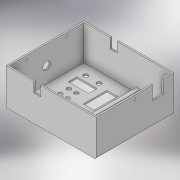
# Autodesk Inventor part: case
Saved by Autodesk Inventor 2019 (Build 230136000, 136)
## iProperties
Created: 2020-05-08
Part Number: case
Material: Generic
Document SubType Name: Modeling
Designer: Mateusz
Density: 1 g/cm^3
Appearance: Default
Author: Mateusz
Autodesk Inventor part; units mm, degrees
ref_plane "YZ Plane" through (0, 0, 0) normal (1, 0, 0) x (0, 1, 0)
ref_plane "XZ Plane" through (0, 0, 0) normal (0, 1, 0) x (-1, 0, 0)
ref_plane "XY Plane" through (0, 0, 0) normal (0, 0, 1) x (1, 0, 0)
sketch "Sketch1" plane through (0, 0, 0) normal (0, 1, 0) x (-1, 0, 0)
  line L0 (0, 0) -> (0, 98.75)
  line L1 (0, 98.75) -> (114.73, 98.75)
  line L2 (114.73, 98.75) -> (114.73, 0)
  line L3 (114.73, 0) -> (0, 0)
  line L4 (0, 98.75) -> (0, 90.47)
  line L5 (0, 0) -> (0, 6.72)
  line L6 (114.73, 0) -> (114.73, 9.87)
  line L7 (-2, 0) -> (-2, 98.75)
  line L8 (-2, 98.75) -> (-2, 100.75)
  line L9 (-2, 100.75) -> (114.73, 100.75)
  line L10 (114.73, 100.75) -> (116.73, 100.75)
  line L11 (116.73, 100.75) -> (116.73, 0)
  line L12 (116.73, 0) -> (116.73, -2)
  line L13 (116.73, -2) -> (-2, -2)
  line L14 (-2, -2) -> (-2, 0)
  dimension "d11" = 2
  dimension "d12" = 2
  dimension "d13" = 2
  dimension "d14" = 2
  constraints: 30 end point, 7 point on line, 6 perpendicular, 1 horizontal, 1 vertical
  measures "d11" distance of L0.start L7.start
  measures "d12" distance of L7.end L8.end
  measures "d13" distance of L9.end L10.end
  measures "d14" distance of L11.end L12.end
extrude "Extrusion1" add sketch "Sketch1" along normal blind 2 contours L0 L1 L2 L3 | L7 L8 L9 L10 L11 L12 L13 L14
extrude "Extrusion9" add sketch "Sketch1" along normal blind 48
sketch "Sketch11" plane through (0, 2, 0) normal (0, 1, 0) x (1, 0, 0)
  circle A0 centre (-60.73, -74.125) radius 3.75 projected
  line L0 (-68.73, -5.5) -> (-68.73, -51.875) projected
  line L1 (-68.73, -5.5) -> (-52.73, -5.5) projected
  line L2 (-68.73, -51.875) -> (-52.73, -51.875) projected
  line L3 (-52.73, -51.875) -> (-52.73, -5.5) projected
  line L4 (-68.53, -92.03) -> (-68.53, -66.625) projected
  line L5 (-68.53, -66.625) -> (-53.65, -66.625) projected
  line L6 (-53.65, -66.625) -> (-53.65, -92.03) projected
  line L7 (-53.65, -92.03) -> (-45.73, -92.03) projected
  line L8 (-45.73, -92.03) -> (-45.73, -5.5) projected
  line L9 (-48.73, -5.5) -> (-45.73, -5.5) projected
  line L10 (-48.73, -5.5) -> (-48.73, -55.875) projected
  line L11 (-48.73, -55.875) -> (-72.73, -55.875) projected
  line L12 (-72.73, -55.875) -> (-72.73, -5.5) projected
  line L13 (-75.73, -5.5) -> (-72.73, -5.5) projected
  line L14 (-75.73, -5.5) -> (-75.73, -17.875) projected
  line L15 (-75.73, -17.875) -> (-85.89, -17.875) projected
  line L16 (-85.89, -17.875) -> (-85.89, -5.5) projected
  line L17 (-85.89, -5.5) -> (-93.51, -5.5) projected
  line L18 (-93.51, -5.5) -> (-93.51, -17.875) projected
  line L19 (-93.51, -17.875) -> (-103.67, -17.875) projected
  line L20 (-103.67, -17.875) -> (-103.67, -5.5) projected
  line L21 (-111.73, -5.5) -> (-103.67, -5.5) projected
  line L22 (-111.73, -5.5) -> (-111.73, -93.25) projected
  line L23 (-111.73, -93.25) -> (-103.67, -93.25) projected
  line L24 (-103.67, -93.25) -> (-103.67, -80.875) projected
  line L25 (-103.67, -80.875) -> (-93.51, -80.875) projected
  line L26 (-93.51, -80.875) -> (-93.51, -92.03) projected
  line L27 (-93.51, -92.03) -> (-85.89, -92.03) projected
  line L28 (-85.89, -92.03) -> (-85.89, -80.875) projected
  line L29 (-85.89, -80.875) -> (-75.73, -80.875) projected
  line L30 (-75.73, -80.875) -> (-75.73, -92.03) projected
  line L31 (-75.73, -92.03) -> (-68.53, -92.03) projected
  line L32 (-56.73, -92.03) -> (-56.73, -81.625) projected
  line L33 (-56.73, -81.625) -> (-64.73, -81.625) projected
  line L34 (-64.73, -81.625) -> (-64.73, -92.03) projected
  line L35 (-64.73, -92.03) -> (-56.73, -92.03) projected
  circle A1 centre (-98.59, -84.875) radius 1.65 projected
  circle A2 centre (-80.81, -84.875) radius 1.65 projected
  circle A3 centre (-60.73, -74.125) radius 3.75 projected
  line L36 (-114.73, -98.25) -> (-114.73, -0.5) projected
  line L37 (-114.73, -0.5) -> (-42.73, -0.5) projected
  line L38 (-42.73, -0.5) -> (-42.73, -98.25) projected
  line L39 (-114.73, -98.25) -> (-42.73, -98.25) projected
  circle A4 centre (-70.73, -23.875) radius 1 projected
  circle A5 centre (-50.73, -23.875) radius 1 projected
  circle A6 centre (-60.73, -53.875) radius 1 projected
  circle A7 centre (-80.81, -13.875) radius 1.65 projected
  circle A8 centre (-98.59, -13.875) radius 1.65 projected
  line L40 (-68.73, -5.5) -> (-68.73, -51.875) projected
  line L41 (-68.73, -51.875) -> (-52.73, -51.875) projected
  line L42 (-52.73, -51.875) -> (-52.73, -5.5) projected
  line L43 (-68.73, -5.5) -> (-52.73, -5.5) projected
  circle A9 centre (-60.73, -74.125) radius 7.5
  line L44 (-67.83, -47.875) -> (-53.63, -47.875)
  line L45 (-67.83, -16.5) -> (-67.83, -47.875)
  line L46 (-53.63, -47.875) -> (-53.63, -16.5)
  line L47 (-53.63, -16.5) -> (-67.83, -16.5)
  line L48 (-42.73, -98.25) -> (-39.73, -98.25)
  line L49 (-39.73, -98.25) -> (-39.73, -0.5)
  line L50 (-39.73, -0.5) -> (-42.73, -0.5)
  line L51 (-42.73, -0.5) -> (-42.73, -98.25)
  circle A10 centre (-96.54, -74.125) radius 3.25
  circle A11 centre (-84.58, -61.395) radius 2.75
  circle A12 centre (-94.53, -61.295) radius 2.75
  circle A13 centre (-94.53, -51.135) radius 2.75
  circle A14 centre (-84.58, -51.395) radius 2.75
  circle A15 centre (-94.53, -40.055) radius 2.75
  circle A16 centre (-84.58, -40.145) radius 2.75
  line L52 (-76.36, -32.405) -> (-103.04, -32.405)
  line L53 (-76.36, -32.405) -> (-76.36, -20.965)
  line L54 (-76.36, -20.965) -> (-103.04, -20.965)
  line L55 (-103.04, -20.965) -> (-103.04, -32.405)
  circle A17 centre (-98.59, -84.875) radius 3
  circle A18 centre (-80.81, -84.875) radius 3
  circle A19 centre (-98.59, -13.875) radius 3
  circle A20 centre (-80.81, -13.875) radius 3
  circle A21 centre (-82.79, -74.125) radius 3.25
  point P0 (0, 0)
  dimension "d49" = 15
  dimension "d56" = 3
  dimension "d109" = 11.44
  dimension "d127" = 6
  dimension "d128" = 6
  dimension "d129" = 6
  dimension "d130" = 6
  dimension "d191" = 6.5
  constraints: 24 end point, 13 centre point, 5 coincident, 4 perpendicular, 2 horizontal, 1 parallel, 1 vertical
  measures "d49" diameter of A9
  measures "d56" distance of L38.end L48.end
  measures "d109" distance of L52.start L53.end
  measures "d127" diameter of A17
  measures "d128" diameter of A18
  measures "d129" diameter of A19
  measures "d130" diameter of A20
  measures "d191" diameter of A21
extrude "Extrusion10" cut sketch "Sketch11" against normal blind 10 contours A0 | A9 L6 | A9 L6 | L45 L47 L46 L44
extrude "Extrusion11" add sketch "Sketch11" along normal blind 7 contours L38 L50 L49 L48
sketch "Sketch12" plane through (-42.73, 2, 0.5) normal (-1, 0, 0) x (0, 0, 1)
  line L0 (97.75, 7) -> (97.75, 5)
  line L1 (97.75, 0) -> (97.75, 7) projected
  line L2 (97.75, 7) -> (0, 7) projected
  line L3 (0, 7) -> (0, 5)
  line L4 (0, 0) -> (0, 7) projected
  line L5 (0, 5) -> (97.75, 5)
  line L6 (97.75, 7) -> (0, 7)
  point P0 (-0.5, -2)
  dimension "d61" = 2
  dimension "d62" = 2
  constraints: 8 end point, 2 point on line
  measures "d61" distance of L0.start L0.end
  measures "d62" distance of L2.end L3.end
extrude "Extrusion12" add sketch "Sketch12" along normal blind 2
extrude "Extrusion13" cut sketch "Sketch11" against normal blind 5 contours A1 | A2 | A7 | A8 | A10 | A11 | A12 | A13 | A14 | A15 | A16 | A21
extrude "Extrusion14" cut sketch "Sketch11" against normal blind 5 contours L52 L55 L54 L53
sketch "Sketch13" plane through (2, 0, 100.75) normal (1, 0, 0) x (0, 0, -1)
  line L0 (88.25, 41) -> (88.75, 41)
  line L1 (88.75, 41) -> (88.75, 48)
  line L2 (88.75, 48) -> (74.75, 48)
  line L3 (74.75, 48) -> (74.75, 41)
  line L4 (74.75, 41) -> (74.75, 30)
  line L5 (74.75, 30) -> (88.5, 30)
  line L6 (88.5, 30) -> (88.75, 30)
  line L7 (88.75, 30) -> (88.75, 41)
  point P0 (100.75, 0)
  point P1 (102.75, 48)
  dimension "d116" = 0.5
  dimension "d118" = 11
  constraints: 16 end point, 3 perpendicular, 2 point on line
  measures "d116" distance of L0.start L0.end
  measures "d118" distance of L3.end L4.end
extrude "Extrusion15" cut sketch "Sketch13" against normal blind 5
sketch "Sketch14" plane through (-116.73, 0, 100.75) normal (0, 0, 1) x (1, 0, 0)
  line L0 (0, 0) -> (0, 48) projected
  line L1 (0, 48) -> (2, 48)
  line L2 (2, 48) -> (36, 48)
  line L3 (2, 48) -> (116.73, 48) projected
  line L4 (36, 48) -> (45, 48)
  line L5 (36, 48) -> (36.715, 48)
  line L6 (0, 48) -> (118.73, 48) projected
  line L7 (36.715, 48) -> (36.715, 35)
  line L8 (45, 48) -> (45.715, 48)
  line L9 (45.715, 48) -> (45.715, 35)
  line L10 (45.715, 35) -> (45, 35)
  line L11 (36.715, 35) -> (45, 35)
  point P0 (116.73, 0)
  dimension "d121" = 2
  dimension "d122" = 34
  dimension "d123" = 9
  dimension "d124" = 13
  dimension "d196" = 0.715
  dimension "d197" = 0.715
  constraints: 18 end point, 4 point on line, 2 perpendicular, 1 collinear, 1 horizontal
  measures "d121" distance of L0.end L1.end
  measures "d122" distance of L1.end L2.end
  measures "d123" distance of L2.end L4.end
  measures "d124" distance of L4.end L10.end
  measures "d196" distance of L2.end L5.end
  measures "d197" distance of L4.end L8.end
extrude "Extrusion16" cut sketch "Sketch14" against normal blind 120
extrude "Extrusion17" add sketch "Sketch11" along normal blind 2 contours A17 | A18 | A19 | A20
sketch "Sketch15" plane through (0, 0, 0) normal (0, -1, 0) x (1, 0, 0)
  line L0 (-2, 12) -> (-2, 26)
  line L1 (-2, 26) -> (-12, 26)
  line L2 (-12, 26) -> (-12, 12)
  line L3 (-12, 12) -> (-2, 12)
  point P0 (0, 0)
  point P1 (2, 12)
  dimension "d134" = 10
  constraints: 8 end point, 3 perpendicular
  measures "d134" distance of L0.end L1.end
extrude "Extrusion18" cut sketch "Sketch15" against normal blind 0.5
sketch "Sketch16" plane through (-116.73, 0, -2) normal (-1, 0, 0) x (0, 0, 1)
  line L0 (2, 48) -> (0, 48) projected
  line L1 (0, 48) -> (20, 48)
  line L2 (100.75, 48) -> (2, 48) projected
  line L3 (20, 48) -> (20, 43)
  line L4 (20, 43) -> (30, 43)
  line L5 (30, 43) -> (25, 43)
  circle A0 centre (25, 43) radius 1.45
  line L6 (102.75, 48) -> (82.75, 48)
  line L7 (28, 48) -> (100.75, 48) projected
  line L8 (82.75, 48) -> (82.75, 43)
  line L9 (82.75, 43) -> (77.75, 43)
  circle A1 centre (77.75, 43) radius 1.45
  point P0 (2, 0)
  dimension "d137" = 20
  dimension "d138" = 5
  dimension "d139" = 10
  dimension "d140" = 2.9
  dimension "d141" = 20
  dimension "d142" = 5
  dimension "d143" = 5
  dimension "d144" = 2.9
  constraints: 14 end point, 3 perpendicular, 2 centre point, 2 coincident, 2 point on line, 1 midpoint, 1 vertical
  measures "d137" distance of L0.end L1.end
  measures "d138" distance of L1.end L3.end
  measures "d139" distance of L3.end L4.end
  measures "d140" diameter of A0
  measures "d141" distance of L6.start L6.end
  measures "d142" distance of L6.end L8.end
  measures "d143" distance of L8.end L9.end
  measures "d144" diameter of A1
extrude "Extrusion19" cut sketch "Sketch16" against normal blind 3
sketch "Sketch17" plane through (2, 0, 100.75) normal (1, 0, 0) x (0, 0, -1)
  circle A0 centre (51.375, 43) radius 1.45
  point P0 (100.75, 0)
  point P1 (0, 48)
  constraints: 1 centre point
extrude "Extrusion20" cut sketch "Sketch17" against normal blind 3
sketch "Sketch18" plane through (0, 0, 0) normal (0, -1, 0) x (1, 0, 0)
  line L0 (-99.53, 40.055) -> (-99.53, 61.295)
  line L1 (-99.53, 61.295) -> (-99.53, 63.795)
  line L2 (-99.53, 63.795) -> (-103.53, 63.795)
  line L3 (-103.53, 63.795) -> (-103.53, 40.055)
  line L4 (-103.53, 40.055) -> (-103.53, 37.555)
  line L5 (-103.53, 37.555) -> (-99.53, 37.555)
  line L6 (-99.53, 37.555) -> (-99.53, 40.055)
  line L7 (-79.58, 61.395) -> (-79.58, 63.895)
  line L8 (-79.58, 63.895) -> (-75.58, 63.895)
  line L9 (-75.58, 63.895) -> (-75.58, 40.055)
  line L10 (-75.58, 40.055) -> (-75.58, 37.555)
  line L11 (-75.58, 37.555) -> (-79.58, 37.555)
  line L12 (-79.58, 37.555) -> (-79.58, 63.895)
  line L13 (-103.04, 20.965) -> (-76.36, 20.965) projected
  line L14 (-103.04, 20.965) -> (-105.04, 20.965)
  line L15 (-105.04, 20.965) -> (-105.04, 32.405)
  line L16 (-103.04, 32.405) -> (-76.36, 32.405) projected
  line L17 (-105.04, 32.405) -> (-109.04, 32.405)
  line L18 (-109.04, 32.405) -> (-109.04, 20.965)
  line L19 (-109.04, 20.965) -> (-105.04, 20.965)
  circle A0 centre (-96.54, 74.125) radius 3.25 projected
  line L20 (-96.54, 74.125) -> (-101.54, 74.125)
  line L21 (-101.54, 74.125) -> (-101.54, 78.125)
  line L22 (-101.54, 78.125) -> (-105.54, 78.125)
  line L23 (-105.54, 78.125) -> (-105.54, 70.125)
  line L24 (-105.54, 70.125) -> (-101.54, 70.125)
  line L25 (-101.54, 70.125) -> (-101.54, 74.125)
  line L26 (-70.73, 74.125) -> (-70.73, 78.125)
  line L27 (-70.73, 78.125) -> (-74.73, 78.125)
  line L28 (-74.73, 78.125) -> (-74.73, 70.125)
  line L29 (-74.73, 70.125) -> (-70.73, 70.125)
  line L30 (-70.73, 74.125) -> (-70.73, 70.125)
  line L31 (-69.83, 47.875) -> (-69.83, 16.5)
  line L32 (-69.83, 16.5) -> (-73.83, 16.5)
  line L33 (-73.83, 16.5) -> (-73.83, 47.875)
  line L34 (-73.83, 47.875) -> (-69.83, 47.875)
  circle A1 centre (-82.79, 74.125) radius 3.25 projected
  line L35 (-82.79, 74.125) -> (-87.79, 74.125)
  line L36 (-87.79, 74.125) -> (-87.79, 78.125)
  line L37 (-87.79, 78.125) -> (-91.79, 78.125)
  line L38 (-91.79, 78.125) -> (-91.79, 70.125)
  line L39 (-91.79, 70.125) -> (-87.79, 70.125)
  line L40 (-87.79, 70.125) -> (-87.79, 74.125)
  point P0 (0, 0)
  point P1 (-94.53, 40.055)
  point P2 (-84.58, 61.395)
  point P3 (-85.81, 74.125)
  point P4 (-85.81, 78.125)
  point P5 (-89.81, 78.125)
  point P6 (-89.81, 70.125)
  point P7 (-85.81, 70.125)
  point P8 (-67.83, 47.875)
  dimension "d153" = 2.5
  dimension "d154" = 4
  dimension "d155" = 2.5
  dimension "d157" = 2.5
  dimension "d158" = 4
  dimension "d159" = 2.5
  dimension "d160" = 4
  dimension "d161" = 2
  dimension "d162" = 4
  dimension "d163" = 5
  dimension "d164" = 4
  dimension "d165" = 4
  dimension "d166" = 8
  dimension "d171" = 4
  dimension "d172" = 4
  dimension "d173" = 8
  dimension "d175" = 4
  dimension "d198" = 5
  dimension "d199" = 4
  dimension "d200" = 8
  constraints: 78 end point, 24 perpendicular, 14 point on line, 2 horizontal, 1 parallel
  measures "d153" distance of L0.end L1.end
  measures "d154" distance of L1.end L2.end
  measures "d155" distance of L3.end L4.end
  measures "d157" distance of L7.start L7.end
  measures "d158" distance of L7.end L8.end
  measures "d159" distance of L9.end L10.end
  measures "d160" distance of L10.end L11.end
  measures "d161" distance of L13.start L14.end
  measures "d162" distance of L15.end L17.end
  measures "d163" distance of L20.start L20.end
  measures "d164" distance of L20.end L21.end
  measures "d165" distance of L21.end L22.end
  measures "d166" distance of L22.end L23.end
  measures "d171" distance of L26.start L26.end
  measures "d172" distance of L26.end L27.end
  measures "d173" distance of L27.end L28.end
  measures "d175" distance of L31.end L32.end
  measures "d198" distance of L35.start L35.end
  measures "d199" distance of L36.end L37.end
  measures "d200" distance of L37.end L38.end
extrude "Extrusion21" cut sketch "Sketch18" against normal blind 0.5 contours L6 L5 L4 L3 L2 L1 L0 | L7 L8 L9 L10 L11 L12 | L19 L18 L17 L15 | A0 | L25 L24 L23 L22 L21 | L30 L29 L28 L27 L26 | L31 L32 L33 L34 | L40 L39 L38 L37 L36
sketch "Sketch19" plane through (0, 0, 0) normal (0, -1, 0) x (1, 0, 0)
  line L0 (-116.73, -2) -> (2, -2) projected
  line L1 (2, -2) -> (2, 8)
  line L2 (2, -2) -> (2, 100.75) projected
  line L3 (2, 8) -> (-18, 8)
  line L4 (2, 100.75) -> (2, 90.75)
  line L5 (2, 90.75) -> (-18, 90.75)
  line L6 (-18, 90.75) -> (-18, 8)
  line L7 (-18, 8) -> (-43, 8)
  line L8 (-43, 8) -> (-43, 90.75)
  line L9 (-43, 90.75) -> (-18, 90.75)
  point P0 (0, 0)
  dimension "d178" = 10
  dimension "d179" = 20
  dimension "d180" = 10
  dimension "d181" = 20
  dimension "d182" = 25
  constraints: 16 end point, 4 perpendicular, 2 point on line, 1 horizontal
  measures "d178" distance of L0.end L1.end
  measures "d179" distance of L1.end L3.end
  measures "d180" distance of L2.end L4.end
  measures "d181" distance of L4.end L5.end
  measures "d182" distance of L3.end L7.end
extrude "Extrusion22" cut sketch "Sketch19" against normal blind 0.5 contours L7 L8 L9 L6
fillet "Fillet1" radius 2 1 edges at (-116.73, 0, 49.375)
sketch "Sketch20" plane through (-116.73, 48, -2) normal (-1, 0, 0) x (0, 0, 1)
  line L0 (100.75, 0) -> (2, 0) projected
  circle A0 centre (51.375, -25) radius 5
  point P0 (2, -48)
  dimension "d187" = 10
  constraints: 1 centre point
  measures "d187" diameter of A0
extrude "Extrusion23" cut sketch "Sketch20" against normal blind 5
sketch "Sketch21" plane through (0, 0, 0) normal (0, -1, 0) x (1, 0, 0)
  circle A0 centre (-98.59, 13.875) radius 1.65 projected
  circle A1 centre (-98.59, 13.875) radius 3
  circle A2 centre (-80.81, 13.875) radius 1.65 projected
  circle A3 centre (-80.81, 13.875) radius 3
  circle A4 centre (-80.81, 84.875) radius 3 projected
  circle A5 centre (-80.81, 84.875) radius 3
  circle A6 centre (-98.59, 84.875) radius 1.65 projected
  circle A7 centre (-98.59, 84.875) radius 3
  point P0 (0, 0)
  dimension "d201" = 6
  dimension "d202" = 6
  dimension "d203" = 6
  dimension "d204" = 6
  constraints: 4 centre point, 4 coincident
  measures "d201" diameter of A1
  measures "d202" diameter of A3
  measures "d203" diameter of A5
  measures "d204" diameter of A7
extrude "Extrusion24" cut sketch "Sketch21" against normal blind 10
body "Solid1"
